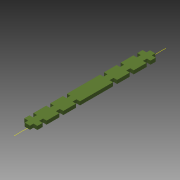
# Autodesk Inventor part: base
Saved by Autodesk Inventor 2015 (Build 190159000, 159)
## iProperties
Created: 2015-12-01
Part Number: base
Material: Generic
Document SubType Name: Modeling
Designer: jufranz
Density: 1 g/cm^3
Appearance: Olive Green
Author: jufranz
Autodesk Inventor part; units mm, degrees
ref_plane "YZ Plane" through (0, 0, 0) normal (1, 0, 0) x (0, 1, 0)
ref_plane "XZ Plane" through (0, 0, 0) normal (0, 1, 0) x (-1, 0, 0)
ref_plane "XY Plane" through (0, 0, 0) normal (0, 0, 1) x (1, 0, 0)
sketch "Sketch1" plane through (0, 0, 0) normal (0, 1, 0) x (-1, 0, 0)
  line L0 (10, 90) -> (-10, 90)
  line L1 (-10, 90) -> (-10, -90)
  line L2 (-10, -90) -> (10, -90)
  line L3 (10, -90) -> (10, 90)
  point P0 (0, 0)
  point P1 (10, 0)
  point P2 (0, 90)
  dimension "d0" = 20
  dimension "d1" = 180
  constraints: 8 end point, 2 midpoint, 2 parallel, 1 horizontal, 1 horizontal alignment, 1 perpendicular, 1 vertical alignment
  measures "d0" distance of L0.start L0.end
  measures "d1" distance of L2.end L0.start
extrude "Extrusion1" add sketch "Sketch1" along normal blind 5.334
sketch "Sketch2" plane through (-10, 0, 90) normal (0, 0, 1) x (1, 0, 0)
  line L0 (0, 5.334) -> (20, 5.334) projected
  line L1 (6, 5.334) -> (14, 5.334)
  line L2 (14, 5.334) -> (14, 0)
  line L3 (14, 0) -> (6, 0)
  line L4 (6, 0) -> (6, 5.334)
  line L5 (0, 0) -> (20, 0) projected
  point P0 (10, 0)
  point P1 (10, 0)
  dimension "d4" = 8
  dimension "d5" = 4
  constraints: 8 end point, 2 midpoint, 2 parallel, 1 horizontal, 1 perpendicular, 1 point on line
  measures "d4" distance between parallel lines of L4 L2
  measures "d5" distance from line of L4 point (10, 0)
extrude "Extrusion2" add sketch "Sketch2" along normal blind 5.334
mirror "Mirror1" about plane through (0, 0, 0) normal (0, 0, 1) of "Extrusion2"
sketch "Sketch3" plane through (10, 0, 90) normal (1, 0, 0) x (0, 0, -1)
  line L0 (0, 5.334) -> (180, 5.334) projected
  line L1 (0, 0) -> (180, 0) projected
  line L2 (8, 5.334) -> (14, 5.334)
  line L3 (14, 5.334) -> (14, 0)
  line L4 (14, 0) -> (8, 0)
  line L5 (8, 0) -> (8, 5.334)
  line L6 (0, 0) -> (0, 5.334) projected
  point P0 (90, 0)
  dimension "d8" = 6
  dimension "d9" = 8
  constraints: 8 end point, 2 parallel, 2 point on line, 1 horizontal, 1 perpendicular
  measures "d8" distance between parallel lines of L3 L5
  measures "d9" distance between parallel lines of L6 L5
extrude "Extrusion3" cut sketch "Sketch3" against normal blind 5.334 contours L0 L3 L1 L5
pattern_linear "Rectangular Pattern1" count 3 spacing 25.4 along (0, 0, -1) of "Extrusion3"
mirror "Mirror2" about plane through (0, 0, 0) normal (0, 0, 1) of "Extrusion3", "Rectangular Pattern1"
mirror "Mirror3" about plane through (0, 0, 0) normal (1, 0, 0) of "Extrusion3", "Rectangular Pattern1", "Mirror2"
equation "\"d5\" = 0.5 * d4"
body "Solid1"
